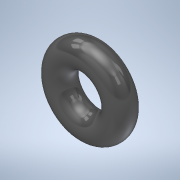
# Autodesk Inventor part: YTP-AP-E05-R1.0
Saved by Autodesk Inventor 2020.4 (Build 244396000, 396)
## iProperties
Created: 2021-08-28
Part Number: YTP-AP-E05-R1.0
Material: Gummi, Silikon
Description: Dichtring-Nadelpackung
Document SubType Name: Modeling
Designer: Uwe Wieser
Mass: 0.0137346 g
Surface Area: 0.351605 cm^2
Volume: 0.0109876 cm^3
Density: 1.25 g/cm^3
Appearance: Gummi - schwarz - Version 1.1
Project: Airbrush
Werkstoff: Gummi
Author: Uwe Wieser
Autodesk Inventor part; units mm, degrees
ref_plane "YZ Plane" through (0, 0, 0) normal (1, 0, 0) x (0, 1, 0)
ref_plane "XZ Plane" through (0, 0, 0) normal (0, 1, 0) x (-1, 0, 0)
ref_plane "XY Plane" through (0, 0, 0) normal (0, 0, 1) x (1, 0, 0)
sketch "Skizze1" plane through (0, 0, 0) normal (0, 0, 1) x (1, 0, 0)
  line L0 (0, -0.875) -> (0, 0.875) projected
  line L1 (-2.87, 0) -> (2.87, 0) projected
  circle A0 centre (-1.425, 0) radius 0.625
  circle A1 centre (1.425, 0) radius 0.625
  point P0 (0, 0)
  dimension "d0" = 1.25
  dimension "d1" = 1.25
  dimension "d4" = 1.6
  constraints: 2 centre point, 2 point on line, 1 symmetric about line
  measures "d0" diameter of A0
  measures "d1" diameter of A1
revolve "Umdrehung1" add sketch "Skizze1" angle 360 about axis through (0, -10, 0) along (0, 1, 0) contours A0 L1 | L1 A0
